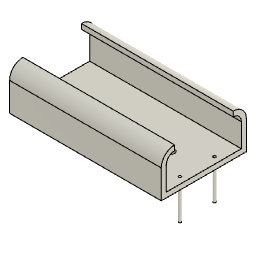
AnhaengerCircuitBox v9 (Autodesk Fusion 360 archive; units mm, degrees)
design "BatterieHalter"
Autodesk Fusion 360 part; units mm, degrees
sketch "Sketch1" plane through (0, 0, 0) normal (0, 0, 1) x (1, 0, 0)
  line L0 (28.5, 16) -> (-28.5, 16)
  line L1 (-28.5, 16) -> (-28.5, -16)
  line L2 (-28.5, -16) -> (28.5, -16)
  line L3 (28.5, -16) -> (28.5, 16)
  line L4 (28.5, 16) -> (-28.5, -16) construction
  line L5 (-28.5, 16) -> (28.5, -16) construction
  circle A0 centre (0, 0) radius 1.65
  circle A1 centre (-7.1, 0) radius 1.4
  line L6 (-28.5, 0) -> (28.5, 0) construction
  circle A2 centre (7.7118, 0) radius 1.4
  circle A3 centre (16.1, 0) radius 1.4
  circle A4 centre (26, 6.5) radius 0.5
  circle A5 centre (26, -6.5) radius 0.5
  line L7 (26, 6.5) -> (26, -6.5) construction
  dimension "d1" = 57
  dimension "d2" = 32
  dimension "d3" = 3.3
  dimension "d4" = 2.8
  dimension "d5" = 7.1
  dimension "d6" = 2.8
  dimension "d7" = 7.7118
  dimension "d8" = 2.8
  dimension "d9" = 16.1
  dimension "d10" = 1
  dimension "d11" = 1
  dimension "d12" = 13
  dimension "d13" = 9.9
  constraint perpendicular L0 L1
  constraint parallel L0 L2
  constraint parallel L1 L3
  constraint horizontal L0
  constraint coincident L4 A0.centre
  constraint coincident L5 A0.centre
  constraint coincident A0.centre origin
  constraint midpoint L1 L6.start
  constraint midpoint L3 L6.end
  constraint coincident A1.centre L6
  constraint coincident L6 A2.centre
  constraint coincident L6 A3.centre
  constraint coincident A4.centre L7.start
  constraint coincident A5.centre L7.end
  constraint vertical L7
  constraint symmetric L6 A4.centre A5.centre
  measures "d1" distance of L1.end L2.end
  measures "d2" distance of L0.end L1.end
  measures "d3" diameter of A0
  measures "d4" diameter of A1
  measures "d5" horizontal distance of A0.centre A1.centre
  measures "d6" diameter of A2
  measures "d7" distance of A0.centre A2.centre
  measures "d8" diameter of A3
  measures "d9" distance of A0.centre A3.centre
  measures "d10" diameter of A4
  measures "d11" diameter of A5
  measures "d12" distance of A4.centre A5.centre
  measures "d13" distance of A3.centre L7
extrude "Extrude1" add sketch "Sketch1" along normal blind 15.7 makes body 1
fillet "Fillet1" radius 5 2 edges at (0, -16, 15.7) (0, 16, 15.7) on bodies 1
sketch "Sketch2" plane through (0, 0, 0) normal (0, 0, -1) x (1, 0, 0)
  circle A0 centre (-7.1, 0) radius 1.4
  circle A1 centre (26, -6.5) radius 0.5
  circle A2 centre (0, 0) radius 1.65
  circle A3 centre (7.7118, 0) radius 1.4
  circle A4 centre (26, 6.5) radius 0.5
  circle A5 centre (16.1, 0) radius 1.4
  line L0 (28.5, -16) -> (28.5, 16)
  line L1 (28.5, 16) -> (-28.5, 16)
  line L2 (-28.5, 16) -> (-28.5, -16)
  line L3 (-28.5, -16) -> (28.5, -16)
  circle A6 centre (26, 6.5) radius 0.5
  circle A7 centre (26, -6.5) radius 0.5
extrude "Extrude2" add sketch "Sketch2" along normal blind 12.8 separate body contours A1 A7 | A4 A6 makes body 2 at (26.1354, -6.9813, -8.5333) makes body 3 at (26.2713, 6.92, -8.5333)
sketch "Sketch3" plane through (28.5, 0, 0) normal (1, 0, 0) x (0, 1, 0)
  arc A0 (16, 10.7) -> (11, 15.7) centre (11, 10.7) ccw
  line L0 (11, 15.7) -> (-11, 15.7)
  arc A1 (-11, 15.7) -> (-16, 10.7) centre (-11, 10.7) ccw
  line L1 (-16, 10.7) -> (-16, 0)
  line L2 (-16, 0) -> (16, 0)
  line L3 (16, 0) -> (16, 10.7)
  line L4 (-14.1, 10.7) -> (-14.1, 1.9)
  line L5 (-14.1, 1.9) -> (14.1, 1.9)
  line L6 (14.1, 1.9) -> (14.1, 10.7)
  arc A2 (14.1, 10.7) -> (11, 13.8) centre (11, 10.7) ccw
  line L7 (11, 13.8) -> (-11, 13.8)
  arc A3 (-11, 13.8) -> (-14.1, 10.7) centre (-11, 10.7) ccw
  dimension "d19" = -1.9
extrude "Extrude3" cut sketch "Sketch3" against normal through all contours L4 L5 L6 A2 L7 A3 bodies 1
sketch "Sketch4" plane through (0, 0, 15.7) normal (0, 0, 1) x (-1, 0, 0)
  circle A0 centre (-16.1, 0) radius 1.4
  circle A1 centre (-26, 6.5) radius 0.5
  circle A2 centre (-7.7118, 0) radius 1.4
  circle A3 centre (0, 0) radius 1.65
  circle A4 centre (-26, -6.5) radius 0.5
  circle A5 centre (7.1, 0) radius 1.4
  line L0 (-28.5, -11) -> (28.5, -11)
  line L1 (28.5, -11) -> (28.5, 11)
  line L2 (28.5, 11) -> (-28.5, 11)
  line L3 (-28.5, 11) -> (-28.5, -11)
  line L4 (28.5, -11) -> (-28.5, -11)
  line L5 (-28.5, 11) -> (28.5, 11)
  line L6 (28.5, -11) -> (28.5, 11)
  line L7 (-28.5, 11) -> (-28.5, -11)
extrude "Extrude4" cut sketch "Sketch4" against normal blind 2 bodies 1
combine "Combine1" operation add target body 3 tool bodies 2 1
